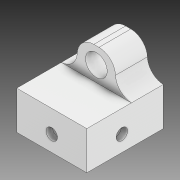
# Autodesk Inventor part: 12110_Shaft Cap_V1
Saved by Autodesk Inventor 2020 (Build 240168000, 168)
## iProperties
Created: 2019-09-27
Part Number: 12110_Shaft Cap_V1
Material: Acetal Resin, White
Document SubType Name: Modeling
Designer: MPI
Density: 1.425 g/cm^3
Appearance: Smooth - White
Author: MPI
Autodesk Inventor part; units mm, degrees
ref_plane "YZ Plane" through (0, 0, 0) normal (1, 0, 0) x (0, 1, 0)
ref_plane "XZ Plane" through (0, 0, 0) normal (0, 1, 0) x (-1, 0, 0)
ref_plane "XY Plane" through (0, 0, 0) normal (0, 0, 1) x (1, 0, 0)
sketch "Sketch1" plane through (0, 0, 0) normal (0, 1, 0) x (-1, 0, 0)
  line L0 (21.5, 22.5) -> (-21.5, 22.5)
  line L1 (-22.5, 21.5) -> (-22.5, -21.5)
  line L2 (-21.5, -22.5) -> (21.5, -22.5)
  line L3 (22.5, -21.5) -> (22.5, 21.5)
  line L4 (27.5, 27.5) -> (-27.5, 27.5)
  line L5 (-27.5, 27.5) -> (-27.5, -27.5)
  line L6 (-27.5, -27.5) -> (27.5, -27.5)
  line L7 (27.5, -27.5) -> (27.5, 27.5)
  arc A0 (22.5, 21.5) -> (21.5, 22.5) centre (22.5, 22.5) ccw
  arc A1 (21.5, -22.5) -> (22.5, -21.5) centre (22.5, -22.5) ccw
  arc A2 (-22.5, -21.5) -> (-21.5, -22.5) centre (-22.5, -22.5) ccw
  arc A3 (-21.5, 22.5) -> (-22.5, 21.5) centre (-22.5, 22.5) ccw
  point P0 (0, 0)
  dimension "d1" = 5
  dimension "d2" = 2
  dimension "d3" = 2
  dimension "d4" = 2
  dimension "d5" = 2
  dimension "d6" = 22.5
  dimension "d7" = 22.5
  dimension "d8" = 45
  constraints: 16 end point, 8 point on circle, 4 centre point, 4 parallel, 3 perpendicular, 1 horizontal
  measures "d1" distance between parallel lines of L3 L7
  measures "d2" diameter of A0
  measures "d3" diameter of A1
  measures "d4" diameter of A2
  measures "d5" diameter of A3
  measures "d6" distance from line of point (0, 0) L3
  measures "d7" distance from line of point (0, 0) L0
  measures "d8" distance between parallel lines of L2 L0
extrude "Extrusion1" add sketch "Sketch1" along normal blind 25
sketch "Sketch2" plane through (0, 25, 0) normal (0, 1, 0) x (1, 0, 0)
  line L0 (-27.5, -27.5) -> (27.5, -27.5)
  line L1 (27.5, -27.5) -> (27.5, 27.5)
  line L2 (27.5, 27.5) -> (-27.5, 27.5)
  line L3 (-27.5, 27.5) -> (-27.5, -27.5)
  line L4 (-27.5, 27.5) -> (-27.5, -27.5) projected
  line L5 (-27.5, -27.5) -> (27.5, -27.5) projected
  line L6 (27.5, 27.5) -> (-27.5, 27.5) projected
  line L7 (27.5, -27.5) -> (27.5, 27.5) projected
  point P0 (0, 0)
  constraints: 8 end point, 4 collinear, 2 parallel, 1 horizontal, 1 perpendicular
extrude "Extrusion2" add sketch "Sketch2" along normal blind 5
sketch "Sketch3" plane through (0, 30, 0) normal (0, 1, 0) x (1, 0, 0)
  line L0 (-27.5, 27.5) -> (-27.5, -27.5) projected
  line L1 (27.5, -27.5) -> (27.5, 27.5) projected
  line L2 (-15, 7.5) -> (15, 7.5)
  line L3 (15, 7.5) -> (15, 27.5)
  line L4 (15, 27.5) -> (-15, 27.5)
  line L5 (-15, 27.5) -> (-15, 7.5)
  line L6 (27.5, 27.5) -> (-27.5, 27.5) projected
  line L7 (-15, 27.5) -> (15, 27.5)
  line L8 (15, 27.5) -> (15, 32.5)
  line L9 (15, 32.5) -> (-15, 32.5)
  line L10 (-15, 32.5) -> (-15, 27.5)
  point P0 (0, 0)
  dimension "d14" = 20
  dimension "d15" = 30
  dimension "d16" = 15
  dimension "d33" = 5
  constraints: 16 end point, 4 parallel, 2 collinear, 2 horizontal, 2 perpendicular
  measures "d14" distance of L4.end L2.start
  measures "d15" distance of L3.end L4.end
  measures "d16" distance from line of point (0, 0) L5
  measures "d33" distance of L9.end L4.end
extrude "Extrusion3" add sketch "Sketch3" along normal blind 25
sketch "Sketch4" plane through (27.5, 0, -27.5) normal (0, 0, -1) x (-1, 0, 0)
  circle A0 centre (27.5, 42) radius 8.5
  line L0 (12.5, 55) -> (42.5, 55) projected
  point P0 (27.5, 0)
  dimension "d19" = 17
  dimension "d20" = 13
  constraints: 1 centre point
  measures "d19" diameter of A0
  measures "d20" distance from line of L0 A0.centre
extrude "Extrusion4" cut sketch "Sketch4" against normal mid plane 40
sketch "Sketch5" plane through (27.5, 0, 27.5) normal (1, 0, 0) x (0, 0, -1)
  circle A0 centre (27.5, 12.5) radius 4.5
  line L0 (0, 0) -> (55, 0) projected
  point P0 (27.5, 0)
  dimension "d25" = 9
  dimension "d26" = 12.5
  constraints: 1 centre point
  measures "d25" diameter of A0
  measures "d26" distance from line of L0 A0.centre
extrude "Extrusion5" cut sketch "Sketch5" against normal through all
sketch "Sketch6" plane through (-27.5, 0, 27.5) normal (0, 0, 1) x (1, 0, 0)
  circle A0 centre (27.5, 12.5) radius 4.5
  point P0 (27.5, 0)
  dimension "d29" = 9
  dimension "d30" = 12.5
  constraints: 1 centre point
  measures "d29" diameter of A0
  measures "d30" distance of point (27.5, 0) A0.centre
extrude "Extrusion6" cut sketch "Sketch6" against normal through all
sketch "Sketch7" plane through (27.5, 0, -27.5) normal (0, 0, -1) x (-1, 0, 0)
  line L0 (0, 30) -> (55, 30)
  line L1 (55, 30) -> (55, 0)
  line L2 (55, 0) -> (0, 0)
  line L3 (0, 0) -> (0, 30)
  line L4 (42.5, 30) -> (55, 30) projected
  line L5 (0, 0) -> (55, 0) projected
  line L6 (55, 0) -> (55, 30) projected
  line L7 (0, 0) -> (0, 30) projected
  circle A0 centre (27.5, 12.5) radius 4.5 projected
  circle A1 centre (27.5, 12.5) radius 4.5
  point P0 (27.5, 0)
  constraints: 8 end point, 4 collinear, 2 parallel, 1 centre point, 1 coincident, 1 horizontal, 1 perpendicular
extrude "Extrusion7" add sketch "Sketch7" along normal blind 5
fillet "Fillet3" radius 13 2 edges at (15, 30, -20) (-15, 30, -20)
fillet "Fillet4" radius 13 2 edges at (-15, 55, -20) (15, 55, -20)
body "Solid1"
